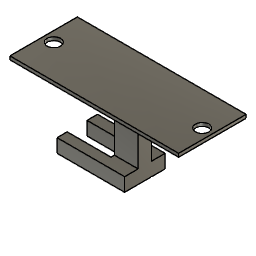
MagnetMountShort (Autodesk Fusion 360 design; units mm, degrees)
Autodesk Fusion 360 part; units mm, degrees
sketch "Sketch1" plane through (0, 0, 0) normal (0, 0, 1) x (1, 0, 0)
  line L0 (0, 0) -> (50, 0)
  line L1 (50, 0) -> (50, 20)
  line L2 (50, 20) -> (0, 20)
  line L3 (0, 20) -> (0, 0)
  dimension "d1" = 50
  dimension "d2" = 20
  constraint horizontal L0
  constraint vertical L1
  constraint horizontal L2
  constraint vertical L3
  constraint coincident L0.start L3.end
  measures "d1" distance of L1.end L2.end
  measures "d2" distance of L0.start L2.end
extrude "Extrude1" add sketch "Sketch1" along normal blind 1
sketch "Sketch2" plane through (0, 0, 1) normal (0, 0, 1) x (-1, 0, 0)
  line L0 (0, -20) -> (0, 0)
  line L1 (0, 0) -> (-50, 0)
  line L2 (-50, 0) -> (-50, -20)
  line L3 (-50, -20) -> (0, -20)
  circle A0 centre (-3, -10) radius 2
  circle A1 centre (-47, -10) radius 2
  dimension "d8" = 4
  dimension "d19" = 4
  measures "d8" diameter of A0
  measures "d19" diameter of A1
extrude "Extrude2" cut sketch "Sketch2" against normal blind 7 contours A0 | A1
sketch "Sketch3" plane through (0, 0, 0) normal (0, 0, -1) x (1, 0, 0)
  circle A0 centre (3, -10) radius 2
  line L0 (0, 0) -> (0, -20)
  line L1 (0, -20) -> (50, -20)
  line L2 (50, -20) -> (50, 0)
  line L3 (50, 0) -> (0, 0)
  line L4 (22.9728, -8) -> (30, -8)
  line L5 (30, -8) -> (30, -12)
  line L6 (30, -12) -> (22.9728, -12)
  line L7 (22.9728, -12) -> (22.9728, -8)
  circle A1 centre (46, -10) radius 2
  circle A2 centre (47, -10) radius 2
  constraint horizontal L4
  constraint vertical L5
  constraint horizontal L6
  constraint vertical L7
extrude "Extrude3" add sketch "Sketch3" along normal blind 21 contours L4 L5 L6 L7
sketch "Sketch6" plane through (0, 8, 0) normal (0, -1, 0) x (1, 0, 0)
  line L0 (30, 0) -> (22.9728, 0)
  line L1 (22.9728, 0) -> (22.9728, -21)
  line L2 (22.9728, -21) -> (30, -21)
  line L3 (30, -21) -> (30, 0)
  line L4 (22.9728, -21) -> (30, -21)
  line L5 (30, -21) -> (30, -17)
  line L6 (30, -17) -> (22.9728, -17)
  line L7 (22.9728, -17) -> (22.9728, -21)
  constraint horizontal L4
  constraint vertical L5
  constraint horizontal L6
  constraint vertical L7
  constraint coincident L3 L5.end
  constraint coincident L1.end L2.start
extrude "Extrude4" add sketch "Sketch6" along normal blind 4 contours L1 L2 L3 L4 L5 L6 L7
extrude "Extrude5" add sketch "Sketch6" against normal blind 8 contours L1 L2 L3 L4 L5 L6 L7
sketch "Sketch7" plane through (22.9728, 0, 0) normal (-1, 0, 0) x (0, -1, 0)
  line L0 (-16, -21) -> (-4, -21)
  line L1 (-4, -21) -> (-4, -17)
  line L2 (-4, -17) -> (-8, -17)
  line L3 (-8, -17) -> (-8, 0)
  line L4 (-8, 0) -> (-12, 0)
  line L5 (-12, 0) -> (-12, -17)
  line L6 (-12, -17) -> (-16, -17)
  line L7 (-16, -17) -> (-16, -21)
  line L8 (-16, -17) -> (-12.8799, -17)
  line L9 (-12.8799, -17) -> (-12.8799, -21)
  line L10 (-12.8799, -21) -> (-16, -21)
  line L11 (-16, -21) -> (-16, -17)
  line L12 (-4, -21) -> (-7, -21)
  line L13 (-7, -21) -> (-7, -17)
  line L14 (-7, -17) -> (-4, -17)
  line L15 (-4, -17) -> (-4, -21)
  constraint horizontal L8
  constraint vertical L9
  constraint horizontal L10
  constraint vertical L11
  constraint coincident L0 L9.end
  constraint coincident L6.end L7.start
  constraint horizontal L12
  constraint vertical L13
  constraint horizontal L14
  constraint vertical L15
  constraint coincident L2 L13.end
  constraint coincident L0.end L1.start
extrude "Extrude6" add sketch "Sketch7" along normal blind 13 contours L0 L6 L7 L8 L9 L10 L11 | L0 L1 L2 L12 L13 L14 L15
